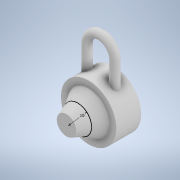
# Autodesk Inventor part: padlock
Saved by Autodesk Inventor 2021 (Build 250183000, 183)
## iProperties
Created: 2022-03-11
Part Number: padlock
Material: Generic
Document SubType Name: Modeling
Designer: User
Density: 1 g/cm^3
Appearance: Default
Author: User
Autodesk Inventor part; units mm, degrees
sketch "Sketch1" plane through (0, 0, 0) normal (0, 0, 1) x (1, 0, 0)
  circle A0 centre (0, 0) radius 10
  dimension "d0" = 20
  constraints: 1 centre point, 1 coincident
  measures "d0" diameter of A0
extrude "Extrusion1" add sketch "Sketch1" along normal blind 9
sketch "Sketch2" plane through (0, 0, 9) normal (0, 0, 1) x (1, 0, 0)
  circle A0 centre (0, 0) radius 7.5
  dimension "d3" = 15
  constraints: 1 centre point, 1 coincident
  measures "d3" diameter of A0
ref_plane "Work Plane1" through (0, 0, 13) normal (0, 0, 1) x (1, 0, 0)
sketch "Sketch3" plane through (0, 0, 13) normal (0, 0, 1) x (1, 0, 0)
  circle A0 centre (0, 0) radius 5
  dimension "d5" = 10
  constraints: 1 centre point, 1 coincident
  measures "d5" diameter of A0
loft "Loft1" add profiles "Sketch2", "Sketch3"
sketch "Sketch4" plane through (0, 0, 13) normal (0, 0, 1) x (1, 0, 0)
  circle A0 centre (0, 0) radius 5
  dimension "d10" = 10
  constraints: 1 centre point, 1 coincident
  measures "d10" diameter of A0
ref_plane "Work Plane2" through (0, 0, 17) normal (0, 0, 1) x (1, 0, 0)
sketch "Sketch5" plane through (0, 0, 17) normal (0, 0, 1) x (1, 0, 0)
  circle A0 centre (0, 0) radius 3.5
  dimension "d12" = 7
  constraints: 1 centre point, 1 coincident
  measures "d12" diameter of A0
loft "Loft2" add profiles "Sketch5" section 1 edges at (-5, 0, 13)
ref_plane "Work Plane3" through (0, 0, 4.5) normal (0, 0, 1) x (1, 0, 0)
sketch "Sketch6" plane through (0, 0, 4.5) normal (0, 0, 1) x (1, 0, 0)
  arc A0 (5, 17) -> (-5.0779, 16.9998) centre (-0.0389, 17) ccw
  line L0 (5, 17) -> (5, 0)
  circle A1 centre (0, 0) radius 5 projected
  line L1 (5, 17) -> (22, 17) construction
  line L2 (-5.0779, 16.9998) -> (-5, 0)
  line L3 (0, 0) -> (0, 5)
  dimension "d20" = 17
  dimension "d21" = 90
  dimension "d22" = 17
  constraints: 8 end point, 4 point on circle, 2 vertical, 1 centre point, 1 horizontal, 1 perpendicular, 1 tangent
  measures "d20" distance of L0.start L0.end
  measures "d21" angle of L0 L1
  measures "d22" distance of L2.start L2.end
ref_plane "Work Plane4" through (5, 0, 4.5) normal (0, -1, 0) x (1, 0, 0)
sketch "Sketch7" plane through (5, 0, 4.5) normal (0, -1, 0) x (1, 0, 0)
  circle A0 centre (0, 0) radius 1.5
  point P0 (-5, -4.5)
  dimension "d23" = 3
  constraints: 1 centre point
  measures "d23" diameter of A0
sweep "Sweep1" add profiles "Sketch7" path "Sketch6" path curves L0 A0 L2
body "Solid1"
